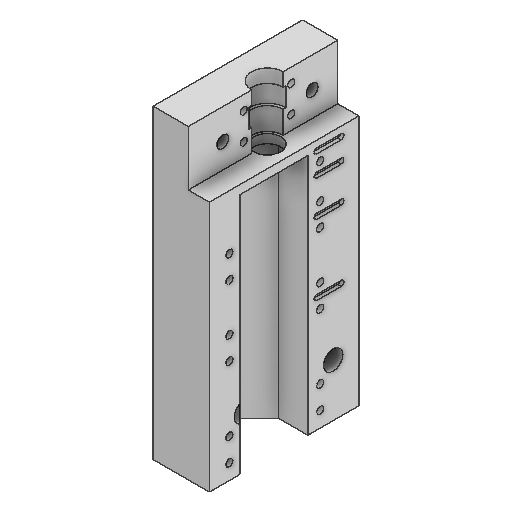
# Autodesk Inventor part: Cuvette Holder Adjustable Transmit
Saved by Autodesk Inventor 2025.1 (Build 291241020, 241B)
## iProperties
Created: 2024-09-19
Part Number: Cuvette Holder Adjustable Transmit
Material: Generic
Document SubType Name: Modeling
Designer: wayneslade
Density: 1 g/cm^3
Appearance: Default
Author: wayneslade
Autodesk Inventor part; units mm, degrees
ref_plane "Work Plane1" through (0, 0, 0) normal (0, 0, 1) x (1, 0, 0)
sketch "Sketch1" plane through (0, 0, 0) normal (0, 0, 1) x (1, 0, 0)
  line L0 (0, 352.2455) -> (0, -445.9232) construction
  line L1 (-20, -9.1281) -> (0, -9.1281)
  line L2 (0, -9.1281) -> (0, -40.3077)
  line L3 (0, -89.1281) -> (-20, -89.1281)
  line L4 (-20, -89.1281) -> (-20, -9.1281)
  line L5 (8.89, -89.1281) -> (-8.89, -89.1281) construction
  line L6 (-18.4, -51.7639) -> (33.4, -51.7639) construction
  line L7 (0, -40.3077) -> (12, -40.3077)
  line L8 (12, -40.3077) -> (12, -63.2201)
  line L9 (12, -63.2201) -> (0, -63.2201)
  line L10 (-8.636, -40.3077) -> (8.636, -40.3077) construction
  line L11 (8.636, -63.2201) -> (-8.636, -63.2201) construction
  line L12 (0, -63.2201) -> (0, -89.1281)
  point P0 (0, 0)
  point P1 (0, -63.2201)
  dimension "d0" = 80
  dimension "d1" = 20
  dimension "d4" = 0
  dimension "d5" = 0
  dimension "d6" = 12
  constraints: 20 end point, 4 parallel, 4 perpendicular, 3 horizontal, 3 point on line, 2 midpoint, 1 collinear, 1 vertical, 4 other
  measures "d0" distance between parallel lines of L1 L3
  measures "d1" distance of L1.start L1.end
  measures "d4" distance between parallel lines of L7 L10
  measures "d5" distance between parallel lines of L11 L9
  measures "d6" distance of L7.start L7.end
extrude "Main Block" add sketch "Sketch1" along normal mid plane 60
ref_plane "Work Plane2" through (0, -51.7639, 0) normal (0, 1, 0) x (0, 0, 1)
ref_plane "Work Plane3" through (-11, -58.2639, -11) normal (0, -1, 0) x (1, 0, 0)
sketch "Sketch3" plane through (0, -51.7639, 0) normal (0, 1, 0) x (0, 0, 1)
  circle A0 centre (0, 0) radius 11 construction
  line L0 (-30, -20) -> (-30, 12) construction
  line L1 (30, 12) -> (30, -20) construction
  line L2 (30, -20) -> (-30, -20) construction
  line L3 (-11, 12) -> (-11, -4.5563)
  line L4 (0, 18.4) -> (0, -26.4) construction
  line L5 (-11, -4.5563) -> (0, -15.5563)
  line L6 (0, -15.5563) -> (27.5563, 12)
  line L7 (-11, 12) -> (27.5563, 12)
  line L8 (-30, 12) -> (30, 12) projected
  point P0 (0, 0)
  dimension "d8" = 90
  constraints: 8 end point, 2 tangent, 1 collinear, 1 parallel, 1 point on line, 1 other
  measures "d8" angle of L6 L5
extrude "Cuvette Cutout" cut sketch "Sketch3" along normal mid plane 12.7
sketch "Sketch4" plane through (0, 0, 0) normal (0, 0, 1) x (1, 0, 0)
  line L0 (-20, -89.1281) -> (-20, -9.1281) construction
  line L1 (-20, -9.1281) -> (0, -9.1281) construction
  line L2 (0, -9.1281) -> (0, -40.3077) construction
  line L3 (0, -40.3077) -> (12, -40.3077) construction
  line L4 (12, -40.3077) -> (12, -45.4139) construction
  line L5 (12, -45.4139) -> (-15.5563, -45.4139) construction
  line L6 (-15.5563, -45.4139) -> (-15.5563, -58.1139) construction
  line L7 (-15.5563, -58.1139) -> (12, -58.1139) construction
  line L8 (12, -63.2201) -> (0, -63.2201) construction
  line L9 (0, -63.2201) -> (0, -89.1281) construction
  line L10 (0, -89.1281) -> (-20, -89.1281) construction
  line L11 (6.3373, -3.5336) -> (6.3373, -4.2956) construction
  line L12 (6.3373, -4.2956) -> (7.2136, -4.2956) construction
  line L13 (7.2136, -4.2956) -> (7.2136, -4.321) construction
  line L14 (7.2136, -4.321) -> (8.2067, -4.321) construction
  spline S0 degree 3 poles (8.2067, -4.321) (8.2067, -4.3168) (8.2067, -4.3125) (8.2067, -4.3041) (8.2067, -4.2998) (8.2067, -4.2956) knots -0.00254 -0.00254 -0.00254 -0.00254 -0.00127 -0.00127 0 0 0 0 construction
  line L15 (8.2067, -4.2956) -> (8.636, -4.2956) construction
  line L16 (8.636, -4.2956) -> (8.89, -4.5496) construction
  line L17 (8.89, -4.5496) -> (8.89, -17.5036) construction
  line L18 (8.89, -17.5036) -> (8.636, -17.7576) construction
  line L19 (8.636, -17.7576) -> (7.0485, -17.7576) construction
  line L20 (7.0485, -17.7576) -> (6.7945, -17.3177) construction
  line L21 (6.7945, -17.3177) -> (6.7945, -5.4386) construction
  line L22 (6.7945, -5.4386) -> (7.1755, -5.4386) construction
  line L23 (7.1755, -5.4386) -> (7.1755, -5.0576) construction
  line L24 (7.1755, -5.0576) -> (5.715, -5.0576) construction
  line L25 (5.715, -5.0576) -> (5.715, -2.5176) construction
  line L26 (5.715, -2.5176) -> (5.969, -2.2636) construction
  line L27 (5.969, -2.2636) -> (6.5405, -2.2636) construction
  line L28 (6.5405, -2.2636) -> (6.7945, -2.7035) construction
  line L29 (6.7945, -2.7035) -> (6.7945, -3.5336) construction
  line L30 (6.7945, -3.5336) -> (6.3373, -3.5336) construction
  line L31 (-7.6987, -4.2956) -> (-7.3452, -4.2956) construction
  spline S1 degree 3 poles (-7.3452, -4.2956) (-7.3452, -4.2998) (-7.3452, -4.3041) (-7.3452, -4.3125) (-7.3452, -4.3168) (-7.3452, -4.321) knots -0.00254 -0.00254 -0.00254 -0.00254 -0.00127 -0.00127 0 0 0 0 construction
  line L32 (-7.3452, -4.321) -> (-7.2079, -4.321) construction
  spline S2 degree 3 poles (-7.2079, -4.321) (-7.2079, -4.3168) (-7.2079, -4.3125) (-7.2079, -4.3041) (-7.2079, -4.2998) (-7.2079, -4.2956) knots -0.00254 -0.00254 -0.00254 -0.00254 -0.00127 -0.00127 0 0 0 0 construction
  line L33 (-7.2079, -4.2956) -> (-6.3373, -4.2956) construction
  line L34 (-6.3373, -4.2956) -> (-6.3373, -3.5336) construction
  line L35 (-6.3373, -3.5336) -> (-6.7945, -3.5336) construction
  line L36 (-6.7945, -3.5336) -> (-6.7945, -2.7035) construction
  line L37 (-6.7945, -2.7035) -> (-6.5405, -2.2636) construction
  line L38 (-6.5405, -2.2636) -> (-5.969, -2.2636) construction
  line L39 (-5.969, -2.2636) -> (-5.715, -2.5176) construction
  line L40 (-5.715, -2.5176) -> (-5.715, -5.0576) construction
  line L41 (-5.715, -5.0576) -> (-7.1755, -5.0576) construction
  line L42 (-7.1755, -5.0576) -> (-7.1755, -5.4386) construction
  line L43 (-7.1755, -5.4386) -> (-6.7945, -5.4386) construction
  line L44 (-6.7945, -5.4386) -> (-6.7945, -17.3177) construction
  line L45 (-6.7945, -17.3177) -> (-7.0485, -17.7576) construction
  line L46 (-7.0485, -17.7576) -> (-8.636, -17.7576) construction
  line L47 (-8.636, -17.7576) -> (-8.89, -17.5036) construction
  line L48 (-8.89, -17.5036) -> (-8.89, -4.5496) construction
  line L49 (-8.89, -4.5496) -> (-8.636, -4.2956) construction
  line L50 (-8.636, -4.2956) -> (-8.2209, -4.2956) construction
  line L51 (-8.2209, -4.2956) -> (-8.2209, -4.321) construction
  line L52 (-8.2209, -4.321) -> (-7.6987, -4.321) construction
  spline S3 degree 3 poles (-7.6987, -4.321) (-7.6987, -4.3168) (-7.6987, -4.3125) (-7.6987, -4.3041) (-7.6987, -4.2998) (-7.6987, -4.2956) knots -0.00254 -0.00254 -0.00254 -0.00254 -0.00127 -0.00127 0 0 0 0 construction
  line L53 (-9.271, -21.089) -> (-9.525, -20.835) construction
  line L54 (-9.525, -20.835) -> (-9.525, -18.549) construction
  line L55 (-9.525, -18.549) -> (-9.271, -18.295) construction
  line L56 (-9.271, -18.295) -> (-7.0485, -18.295) construction
  line L57 (-7.0485, -18.295) -> (-6.7945, -18.7349) construction
  line L58 (-6.7945, -18.7349) -> (-6.7945, -20.6491) construction
  line L59 (-6.7945, -20.6491) -> (-7.0485, -21.089) construction
  line L60 (-7.0485, -21.089) -> (-9.271, -21.089) construction
  line L61 (9.525, -20.835) -> (9.271, -21.089) construction
  line L62 (9.271, -21.089) -> (7.0485, -21.089) construction
  line L63 (7.0485, -21.089) -> (6.7945, -20.6491) construction
  line L64 (6.7945, -20.6491) -> (6.7945, -18.7349) construction
  line L65 (6.7945, -18.7349) -> (7.0485, -18.295) construction
  line L66 (7.0485, -18.295) -> (9.271, -18.295) construction
  line L67 (9.271, -18.295) -> (9.525, -18.549) construction
  line L68 (9.525, -18.549) -> (9.525, -20.835) construction
  line L69 (6.096, -26.0837) -> (6.096, -26.8457) construction
  line L70 (6.096, -26.8457) -> (8.636, -26.8457) construction
  line L71 (8.636, -26.8457) -> (8.89, -27.0997) construction
  line L72 (8.89, -27.0997) -> (8.89, -40.0537) construction
  line L73 (8.89, -40.0537) -> (8.636, -40.3077) construction
  line L74 (8.636, -40.3077) -> (8.3609, -40.3077) construction
  spline S4 degree 3 poles (8.3609, -40.3077) (8.3609, -40.3073) (8.3609, -40.3068) (8.3609, -40.306) (8.3609, -40.3056) (8.3609, -40.3052) knots -0.000254 -0.000254 -0.000254 -0.000254 -0.000127 -0.000127 0 0 0 0 construction
  line L75 (8.3609, -40.3052) -> (7.239, -40.3052) construction
  spline S5 degree 3 poles (7.239, -40.3052) (7.239, -40.3056) (7.239, -40.306) (7.239, -40.3068) (7.239, -40.3073) (7.239, -40.3077) knots -0.000254 -0.000254 -0.000254 -0.000254 -0.000127 -0.000127 0 0 0 0 construction
  line L76 (7.239, -40.3077) -> (7.0485, -40.3077) construction
  line L77 (7.0485, -40.3077) -> (6.7945, -39.8678) construction
  line L78 (6.7945, -39.8678) -> (6.7945, -27.9887) construction
  line L79 (6.7945, -27.9887) -> (7.112, -27.9887) construction
  line L80 (7.112, -27.9887) -> (7.112, -27.6077) construction
  line L81 (7.112, -27.6077) -> (5.715, -27.6077) construction
  line L82 (5.715, -27.6077) -> (5.715, -14.1457) construction
  line L83 (5.715, -14.1457) -> (6.5405, -14.1457) construction
  line L84 (6.5405, -14.1457) -> (6.7945, -14.5856) construction
  line L85 (6.7945, -14.5856) -> (6.7945, -26.0837) construction
  line L86 (6.7945, -26.0837) -> (6.096, -26.0837) construction
  line L87 (-7.428, -40.3077) -> (-7.8325, -40.3077) construction
  spline S6 degree 3 poles (-7.8325, -40.3077) (-7.8325, -40.3073) (-7.8325, -40.3068) (-7.8325, -40.306) (-7.8325, -40.3056) (-7.8325, -40.3052) knots -0.000254 -0.000254 -0.000254 -0.000254 -0.000127 -0.000127 0 0 0 0 construction
  line L88 (-7.8325, -40.3052) -> (-8.3387, -40.3052) construction
  line L89 (-8.3387, -40.3052) -> (-8.3387, -40.3077) construction
  line L90 (-8.3387, -40.3077) -> (-8.636, -40.3077) construction
  line L91 (-8.636, -40.3077) -> (-8.89, -40.0537) construction
  line L92 (-8.89, -40.0537) -> (-8.89, -27.0997) construction
  line L93 (-8.89, -27.0997) -> (-8.636, -26.8457) construction
  line L94 (-8.636, -26.8457) -> (-6.096, -26.8457) construction
  line L95 (-6.096, -26.8457) -> (-6.096, -26.0837) construction
  line L96 (-6.096, -26.0837) -> (-6.7945, -26.0837) construction
  line L97 (-6.7945, -26.0837) -> (-6.7945, -14.5856) construction
  line L98 (-6.7945, -14.5856) -> (-6.5405, -14.1457) construction
  line L99 (-6.5405, -14.1457) -> (-5.715, -14.1457) construction
  line L100 (-5.715, -14.1457) -> (-5.715, -27.6077) construction
  line L101 (-5.715, -27.6077) -> (-7.112, -27.6077) construction
  line L102 (-7.112, -27.6077) -> (-7.112, -27.9887) construction
  line L103 (-7.112, -27.9887) -> (-6.7945, -27.9887) construction
  line L104 (-6.7945, -27.9887) -> (-6.7945, -39.8678) construction
  line L105 (-6.7945, -39.8678) -> (-7.0485, -40.3077) construction
  line L106 (-7.0485, -40.3077) -> (-7.3053, -40.3077) construction
  spline S7 degree 3 poles (-7.3053, -40.3077) (-7.3053, -40.3073) (-7.3053, -40.3068) (-7.3053, -40.306) (-7.3053, -40.3056) (-7.3053, -40.3052) knots -0.000254 -0.000254 -0.000254 -0.000254 -0.000127 -0.000127 0 0 0 0 construction
  line L107 (-7.3053, -40.3052) -> (-7.428, -40.3052) construction
  spline S8 degree 3 poles (-7.428, -40.3052) (-7.428, -40.3056) (-7.428, -40.306) (-7.428, -40.3068) (-7.428, -40.3073) (-7.428, -40.3077) knots -0.000254 -0.000254 -0.000254 -0.000254 -0.000127 -0.000127 0 0 0 0 construction
  line L108 (-8.95, -8.1281) -> (-8.95, -16.7529)
  line L109 (-8.95, -16.7529) -> (-10.525, -16.7529)
  line L110 (-10.525, -16.7529) -> (-10.525, -27.6597)
  line L111 (-10.525, -27.6597) -> (-8.95, -27.6597)
  line L112 (-8.95, -27.6597) -> (-8.95, -40.3052)
  line L113 (-20, -9.1281) -> (0, -9.1281) construction
  line L114 (-5.5245, -76.2329) -> (-5.5245, -31.3309) construction
  arc A0 (-5.5245, -31.3309) -> (5.5245, -31.3309) centre (0, 12.4923) ccw construction
  line L115 (5.5245, -31.3309) -> (5.5245, -76.2329) construction
  line L116 (-7.5245, -40.3052) -> (-7.5245, -45.4139)
  line L117 (-8.95, -40.3052) -> (-7.5245, -40.3052)
  line L118 (-7.5245, -45.4139) -> (0, -45.4139)
  line L119 (0, -45.4139) -> (0, -8.1281)
  line L120 (0, -8.1281) -> (-8.95, -8.1281)
  line L121 (12, -58.1139) -> (12, -63.2201) projected
  point P0 (0, 0)
  dimension "d12" = 1
  dimension "d14" = 0
  dimension "d16" = 1
  dimension "d73" = 1.4255
  dimension "d74" = 2
  dimension "d138" = 0.06
  dimension "d139" = 0.06
  constraints: 218 end point, 40 horizontal, 33 vertical, 9 perpendicular, 9 vertical alignment, 2 collinear, 2 point on circle, 1 centre point, 1 parallel, 156 other
  measures "d12" distance between parallel lines of L110 L54
  measures "d14" distance between parallel lines of L117 L88
  measures "d16" distance between parallel lines of L120 L1
  measures "d73" distance of L112.end L116.start
  measures "d74" distance between parallel lines of L116 L114
  measures "d138" distance between parallel lines of L108 L48
  measures "d139" distance between parallel lines of L112 L92
revolve "Lens Tubes Cutout" cut sketch "Sketch4" angle 360 about axis through (0, -45.4139, 0) along (0, 1, 0)
sketch "Sketch8" plane through (0, 0, 30) normal (0, 0, 1) x (1, 0, 0)
  line L0 (-20, -89.1281) -> (0, -89.1281) projected
  line L1 (0, -89.1281) -> (0, -63.2201) projected
  line L2 (0, -63.2201) -> (12, -63.2201) projected
  line L3 (12, -63.2201) -> (12, -40.3077) projected
  line L4 (12, -40.3077) -> (0, -40.3077) projected
  line L5 (0, -40.3077) -> (0, -9.1281) projected
  line L6 (0, -9.1281) -> (-20, -9.1281) projected
  line L7 (-20, -9.1281) -> (-20, -89.1281) projected
  point P0 (0, 0)
extrude "Extend Base Front" add sketch "Sketch8" along normal blind 15
sketch "Sketch9" plane through (0, 0, -30) normal (0, 0, -1) x (-1, 0, 0)
  line L0 (0, -89.1281) -> (20, -89.1281) projected
  line L1 (20, -89.1281) -> (20, -9.1281) projected
  line L2 (20, -9.1281) -> (0, -9.1281) projected
  line L3 (0, -9.1281) -> (0, -40.3077) projected
  line L4 (0, -40.3077) -> (-12, -40.3077) projected
  line L5 (-12, -40.3077) -> (-12, -63.2201) projected
  line L6 (-12, -63.2201) -> (0, -63.2201) projected
  line L7 (0, -63.2201) -> (0, -89.1281) projected
  point P0 (0, 0)
extrude "Extend Base Back" add sketch "Sketch9" along normal blind 10
sketch "Sketch12" plane through (0, -63.2201, 45) normal (0, -1, 0) x (1, 0, 0)
  line L0 (12, -85) -> (12, 0) projected
  line L1 (-20, -85) -> (-20, 0) projected
  line L2 (12, 0) -> (-20, 0)
  line L3 (-20, 0) -> (-20, -85)
  line L4 (-20, -85) -> (12, -85)
  line L5 (12, -85) -> (12, 0)
  point P0 (0, -45)
  constraints: 8 end point, 2 parallel, 1 horizontal, 1 perpendicular
extrude "Extend Block For Adjustable" add sketch "Sketch12" along normal blind 120
sketch "Sketch13" plane through (0, -58.1139, 0) normal (0, 1, 0) x (1, 0, 0)
  line L0 (-4.5563, 11) -> (12, 11) projected
  line L1 (-15.5563, 0) -> (-4.5563, 11) projected
  line L2 (12, -27.5563) -> (-15.5563, 0) projected
  line L3 (12, 11) -> (12, -27.5563) projected
  point P0 (0, 0)
extrude "Extend Cuvette Cutout" cut sketch "Sketch13" against normal through all
sketch "Sketch10" plane through (-20, -89.1281, 45) normal (-1, 0, 0) x (0, 0, 1)
  line L0 (-45, 120.4765) -> (-45, -98.9624) construction
  line L1 (-102, 37.3642) -> (17, 37.3642) construction
  circle A0 centre (-19.6, 62.7642) radius 3.3782
  circle A1 centre (-19.6, -64.2358) radius 3.3782
  circle A2 centre (-70.4, 62.7642) radius 3.3782
  circle A3 centre (-70.4, -64.2358) radius 3.3782
  point P0 (-45, 89.1281)
  point P1 (-45, 37.3642)
  dimension "d102" = 6.7564
  dimension "d105" = 25.4
  dimension "d106" = 25.4
  dimension "d107" = 6.7564
  dimension "d108" = 25.4
  dimension "d109" = 101.6
  constraints: 4 centre point, 2 point on line, 2 symmetric about line, 2 other
  measures "d102" diameter of A0
  measures "d105" horizontal distance of point (-45, 37.364) A0.centre
  measures "d106" horizontal distance of point (-45, 37.364) A0.centre
  measures "d107" diameter of A1
  measures "d108" distance from line of L0 A1.centre
  measures "d109" vertical distance of A1.centre point (-45, 37.364)
extrude "Breadboard Holes" cut sketch "Sketch10" against normal through all
sketch "Sketch17" plane through (12, -45.4139, 27.5563) normal (1, 0, 0) x (0, 0, -1)
  circle A0 centre (52.9563, -107.95) radius 3.3782 construction
  circle A1 centre (52.9563, -107.95) radius 3.3782 construction
  arc A2 (0, -110.5505) -> (0, -105.3495) centre (2.1563, -107.95) ccw construction
  arc A3 (0, -105.3495) -> (0, -110.5505) centre (2.1563, -107.95) ccw construction
  circle A4 centre (2.1563, -107.95) radius 3.3782 construction
  circle A5 centre (52.9563, -107.95) radius 5.5
  circle A6 centre (2.1563, -107.95) radius 5.5
  point P0 (27.5563, 45.4139)
  dimension "d110" = 11
  dimension "d111" = 11
  constraints: 2 centre point, 2 coincident
  measures "d110" diameter of A5
  measures "d111" diameter of A6
extrude "Counterbore Breadboard Holes" cut sketch "Sketch17" against normal up to surface (12 mm away)
sketch "Sketch15" plane through (12, -45.4139, 27.5563) normal (1, 0, 0) x (0, 0, -1)
  line L0 (-4.35, -131.5) -> (-4.35, -126.5) construction
  arc A0 (-4.35, -126.5) -> (-7.85, -126.5) centre (-6.1, -126.5) ccw construction
  line L1 (-7.85, -126.5) -> (-7.85, -131.5) construction
  arc A1 (-7.85, -131.5) -> (-4.35, -131.5) centre (-6.1, -131.5) ccw construction
  line L2 (-4.35, -118.5) -> (-4.35, -113.5) construction
  arc A2 (-4.35, -113.5) -> (-7.85, -113.5) centre (-6.1, -113.5) ccw construction
  line L3 (-7.85, -113.5) -> (-7.85, -118.5) construction
  arc A3 (-7.85, -118.5) -> (-4.35, -118.5) centre (-6.1, -118.5) ccw construction
  line L4 (-13.4437, -107.5) -> (-13.4437, -137.5) construction
  line L5 (0.9, -107.5) -> (0.9, -137.5) construction
  line L6 (84.5563, -102.5) -> (-34.4437, -102.5) construction
  line L7 (84.5563, -52.5) -> (-34.4437, -52.5) construction
  line L8 (84.5563, -12.5) -> (-34.4437, -12.5) construction
  line L9 (-13.4437, -107.5) -> (0.9, -107.5) projected
  line L10 (-6.1, -138.1825) -> (-6.1, -12.5) construction
  line L11 (19.7282, -102.5) -> (19.7282, -137.5) construction
  line L12 (-4.35, -113.5) -> (-7.85, -118.5) construction
  line L13 (-4.35, -126.5) -> (-7.85, -131.5) construction
  line L14 (-13.4437, -137.5) -> (0.9, -137.5) projected
  point P0 (27.5563, 45.4139)
  point P1 (-16.4437, -102.5)
  point P2 (0.9, -102.5)
  point P3 (38.5563, -102.5)
  point P4 (55.9, -102.5)
  point P5 (-6.1, -116)
  point P6 (-6.1, -129)
  point P7 (-6.1, -66)
  point P8 (-6.1, -79)
  point P9 (-6.1, -26)
  point P10 (-6.1, -39)
  point P11 (45.5563, -116)
  point P12 (45.5563, -129)
  point P13 (45.5563, -66)
  point P14 (45.5563, -79)
  point P15 (45.5563, -26)
  point P16 (45.5563, -39)
  dimension "d84" = 13.5
  dimension "d85" = 13
  dimension "d86" = 13.5
  dimension "d87" = 13
  dimension "d88" = 13.5
  dimension "d89" = 13
  constraints: 12 end point, 6 point on line, 6 symmetric about line, 3 horizontal, 2 midpoint, 1 parallel, 1 perpendicular, 6 other
  measures "d84" distance from line of point (-6.1, -116) L6
  measures "d85" distance of point (-6.1, -129) point (-6.1, -116)
  measures "d86" distance from line of point (-6.1, -66) L7
  measures "d87" distance of point (-6.1, -79) point (-6.1, -66)
  measures "d88" distance from line of point (-6.1, -26) L8
  measures "d89" distance of point (-6.1, -39) point (-6.1, -26)
hole "Holes for Rcv Holddown M3 Inserts" at (12, -161.4139, 33.6563) at (12, -174.4139, 33.6563) at (12, -111.4139, 33.6563) at (12, -124.4139, 33.6563) at (12, -71.4139, 33.6563) at (12, -84.4139, 33.6563) at (12, -71.4139, -18) at (12, -84.4139, -18) at (12, -111.4139, -18) at (12, -124.4139, -18) at (12, -161.4139, -18) at (12, -174.4139, -18) direction (-1, 0, 0) diameter 4 depth 10
sketch "Sketch20" plane through (0, -40.3077, 0) normal (0, 1, 0) x (1, 0, 0)
  arc A0 (0, -7.5245) -> (0, 7.5245) centre (0, 0) ccw projected
  line L0 (0, -7.5245) -> (0, -45) projected
  line L1 (12, -45) -> (0, -45) projected
  line L2 (12, 40) -> (12, -45) projected
  line L3 (0, 40) -> (12, 40) projected
  line L4 (0, 40) -> (0, 7.5245) projected
  line L5 (0, 8.95) -> (0, 7.5245) projected
  arc A1 (0, 8.95) -> (0, -8.95) centre (0, 0) ccw projected
  line L6 (0, -7.5245) -> (0, -8.95) projected
  arc A2 (0, 7.5245) -> (0, -7.5245) centre (0, 0) ccw projected
  point P0 (0, 0)
  point P1 (0, -8.95)
  point P2 (0, 8.95)
extrude "Trim Transmit Bulkhead to 5mm" cut sketch "Sketch20" along normal blind 0.1 and the other way blind 0.106 contours A0 L4 L3 L2 L1 L0 | L0 A1 L4 A2
sketch "Sketch21" plane through (0, -27.6597, 10.525) normal (1, 0, 0) x (0, 0, -1)
  circle A0 centre (-2.975, 10.5316) radius 1.75 construction
  circle A1 centre (-2.975, -4.754) radius 1.75 construction
  circle A2 centre (24.025, -4.754) radius 1.75 construction
  circle A3 centre (24.025, 10.5316) radius 1.75 construction
  point P0 (10.525, 27.6597)
  constraints: 3 centre point, 6 other
hole "Holes for Trans Holddown M3 Inserts" at (0, -17.1281, 13.5) at (0, -32.4137, 13.5) at (0, -32.4137, -13.5) at (0, -17.1281, -13.5) direction (-1, 0, 0) diameter 4 depth 10
sketch "Sketch5" plane through (12, -63.2201, 30) normal (1, 0, 0) x (0, 0, -1)
  line L0 (60, 11.5562) -> (41, 11.5562) construction
  line L1 (41, 13.9562) -> (41, 8.9562)
  line L2 (67.0766, 5.5562) -> (41, 5.5562) construction
  line L3 (60, -80.0818) -> (60, 22.9228) construction
  line L4 (46, -81.4007) -> (46, 22.5472) construction
  line L5 (46, 5.5562) -> (60, 5.5562) construction
  line L6 (46, 4.0562) -> (60, 4.0562)
  line L7 (60, 7.0562) -> (46, 7.0562)
  arc A0 (46, 7.0562) -> (46, 4.0562) centre (46, 5.5562) ccw
  arc A1 (60, 4.0562) -> (60, 7.0562) centre (60, 5.5562) ccw
  line L8 (46, 19.0562) -> (60, 19.0562)
  line L9 (60, 16.0562) -> (46, 16.0562)
  arc A2 (46, 19.0562) -> (46, 16.0562) centre (46, 17.5562) ccw
  arc A3 (60, 16.0562) -> (60, 19.0562) centre (60, 17.5562) ccw
  line L10 (41, 5.3062) -> (19, 5.3062) construction
  line L11 (41, 17.8062) -> (19, 17.8062) construction
  line L12 (41, 5.3062) -> (41, 17.8062) construction
  line L13 (14.6, 11.5562) -> (45.4, 11.5562) construction
  line L14 (65.9522, 0.3062) -> (43.1094, 0.3062) construction
  line L15 (70, 22.8064) -> (70, -120) construction
  circle A4 centre (48, -8.1938) radius 2 construction
  circle A5 centre (48, -21.1938) radius 2 construction
  circle A6 centre (48, -48.1938) radius 2 construction
  circle A7 centre (48, -61.1938) radius 2 construction
  line L16 (48, -8.1938) -> (48, -21.1938) construction
  line L17 (48, -48.1938) -> (48, -61.1938) construction
  line L18 (46, -14.6938) -> (60, -14.6938) construction
  line L19 (46, -16.1938) -> (60, -16.1938)
  line L20 (60, -13.1938) -> (46, -13.1938)
  arc A8 (46, -13.1938) -> (46, -16.1938) centre (46, -14.6938) ccw
  arc A9 (60, -16.1938) -> (60, -13.1938) centre (60, -14.6938) ccw
  line L21 (46, -54.6938) -> (60, -54.6938) construction
  line L22 (46, -56.1938) -> (60, -56.1938)
  line L23 (60, -53.1938) -> (46, -53.1938)
  arc A10 (46, -53.1938) -> (46, -56.1938) centre (46, -54.6938) ccw
  arc A11 (60, -56.1938) -> (60, -53.1938) centre (60, -54.6938) ccw
  point P0 (30, 63.2201)
  point P1 (50.5, 17.5562)
  point P2 (53, 5.5562)
  point P3 (48, -14.6938)
  point P4 (48, -54.6938)
  point P5 (53, -14.6938)
  point P6 (53, -54.6938)
  dimension "d30" = 6
  dimension "d31" = 6
  dimension "d131" = 5
  dimension "d132" = 5
  dimension "d133" = 10
  dimension "d135" = 3
  dimension "d136" = 3
  dimension "d137" = 3
  constraints: 48 end point, 16 point on circle, 12 tangent, 10 point on line, 8 centre point, 6 symmetric about line, 5 midpoint, 5 parallel, 4 perpendicular, 3 vertical, 2 horizontal, 1 collinear, 4 other
  measures "d30" distance between parallel lines of L0 L2
  measures "d31" distance from line of point (50.5, 17.556) L0
  measures "d131" distance between parallel lines of L14 L10
  measures "d132" distance between parallel lines of L12 L4
  measures "d133" distance between parallel lines of L15 L3
  measures "d135" distance between parallel lines of L19 L20
  measures "d136" distance between parallel lines of L6 L7
  measures "d137" distance between parallel lines of L22 L23
extrude "Slots for Cuvette Aligners" cut sketch "Sketch5" against normal blind 2
sketch "Sketch6" plane through (12, -63.2201, 30) normal (1, 0, 0) x (0, 0, -1)
  circle A0 centre (48, -8.1938) radius 2 construction
  circle A1 centre (48, -21.1938) radius 2 construction
  line L0 (48, 22.1251) -> (48, -56.6234) construction
  line L1 (60, 16.0562) -> (46, 16.0562) construction
  line L2 (46, 7.0562) -> (60, 7.0562) construction
  line L3 (14.6, 11.5562) -> (45.4, 11.5562) construction
  line L4 (45.4, 11.5562) -> (48, 11.5562) construction
  point P0 (30, 63.2201)
  constraints: 6 end point, 3 point on line, 1 horizontal, 1 perpendicular, 2 other
hole "Hole for 10mm Cuvette Aligner M3 Insert" at (12, -51.6639, -18) direction (-1, 0, 0) diameter 4 depth 8 tip angle 118
equation "\"d107\" = d102"
equation "\"d108\" = d105"
equation "\"d111\" = d110"
equation "\"d86\" = d84"
equation "\"d87\" = d85"
equation "\"d88\" = d84"
equation "\"d89\" = d85"
equation "\"d31\" = d30"
body "Solid1"
